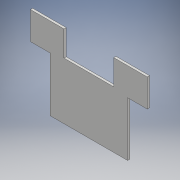
# Autodesk Inventor part: 床板
Saved by Autodesk Inventor 2018 (Build 220112000, 112)
## iProperties
Created: 2017-10-09
Part Number: 床板
Material: 一般
Document SubType Name: Modeling
Designer: Kosei
Density: 1 g/cm^3
Appearance: 既定
Author: Kosei
Autodesk Inventor part; units mm, degrees
ref_plane "YZ Plane" through (0, 0, 0) normal (1, 0, 0) x (0, 1, 0)
ref_plane "XZ Plane" through (0, 0, 0) normal (0, 1, 0) x (-1, 0, 0)
ref_plane "XY Plane" through (0, 0, 0) normal (0, 0, 1) x (1, 0, 0)
sketch "スケッチ1" plane through (0, 0, 0) normal (0, 1, 0) x (-1, 0, 0)
  line L0 (-640, 0) -> (-640, -304.5333)
  line L1 (-425, -900) -> (425, -900)
  line L2 (640, -304.5333) -> (640, 0)
  line L3 (-272.8, 0) -> (-272.8, -277.3333)
  line L4 (-272.8, -277.3333) -> (272.8, -277.3333)
  line L5 (272.8, -277.3333) -> (272.8, 0)
  line L6 (0, -900) -> (0, 0) construction
  line L7 (640, 0) -> (272.8, 0)
  line L8 (-272.8, 0) -> (-640, 0)
  line L9 (-425, -900) -> (-425, -304.5333)
  line L10 (-425, -304.5333) -> (-640, -304.5333)
  line L11 (640, -277.3333) -> (640, -304.5333)
  line L12 (-425, -304.5333) -> (640, -304.5333) construction
  line L13 (640, -304.5333) -> (425, -304.5333)
  line L14 (425, -304.5333) -> (425, -900)
  point P0 (0, 0)
  dimension "d4" = 545.6
  dimension "d5" = 622.6667
  dimension "d9" = 215
  dimension "d10" = 595.4667
  dimension "d14" = 1280
  dimension "d15" = 900
  dimension "d16" = 367.2
  dimension "d17" = 304.5333
  dimension "d18" = 850
  constraints: 30 end point, 7 horizontal, 5 perpendicular, 4 parallel, 1 midpoint, 4 other
  measures "d4" distance of L3.end L4.end
  measures "d5" distance between parallel lines of L4 L1
  measures "d9" distance of L0.end L9.end
  measures "d10" distance of L1.start L9.end
  measures "d14" distance between parallel lines of L0 L2
  measures "d15" distance between parallel lines of L8 L1
  measures "d16" distance of L3.start L0.start
  measures "d17" distance of L0.start L0.end
  measures "d18" distance of L1.start L1.end
extrude "押し出し1" add sketch "スケッチ1" along normal blind 25
